Test Fit 2 mm new sketch design from OS 7 1_v1 (Autodesk Fusion 360 design; units mm, degrees)
Autodesk Fusion 360 part; units mm, degrees
(part 1 of 2)
ref_plane "WorkPlane12" through (0, -1, 0) normal (0, 1, 0) x (0, 0, 1)
sketch "MyStock" plane through (0, 0, 0) normal (0, 0, 1) x (1, 0, 0)
  line L0 (-9.525, 182) -> (9.525, 182)
  line L1 (9.525, 182) -> (9.525, 0)
  line L2 (-9.525, 0) -> (-9.525, 182)
  line L3 (-9.525, 0) -> (9.525, 0)
  dimension "d2016" = 9.525
  dimension "d2017" = 9.525
  dimension "d2102" = 182
  constraint horizontal L0
  constraint vertical L1
  constraint vertical L2
  constraint perpendicular L1 L3
  constraint coincident origin L3
  measures "d2016" distance of origin L1
  measures "d2017" distance of origin L2
  measures "d2102" vertical distance of origin L0.end
extrude "Extrude21" add sketch "MyStock" along normal blind 3.175 makes body 1
sketch "Box Big part" plane through (0, 0, 0) normal (0, 0, 1) x (1, 0, 0)
  line L0 (-224.905, 0) -> (-240, 0)
  line L1 (0, 16.095) -> (0, 0)
  line L2 (-240, 0) -> (-224.905, 0)
  line L3 (-224.905, 0) -> (-224.905, 1.5613)
  line L4 (-223.7758, 3.175) -> (-216.2242, 3.175)
  line L5 (-215.095, 1.5613) -> (-215.095, 0)
  line L6 (-240, 16.095) -> (-238.4387, 16.095)
  line L7 (-236.825, 17.2242) -> (-236.825, 24.7758)
  line L8 (-238.4387, 25.905) -> (-240, 25.905)
  line L9 (-215.095, 0) -> (-204.905, 0)
  line L10 (1.75, 0) -> (22.5, 0)
  arc A0 (-215.095, 1.5613) -> (-216.2242, 3.175) centre (-215.5171, 2.4679) ccw
  arc A1 (-223.7758, 3.175) -> (-224.905, 1.5613) centre (-224.4829, 2.4679) ccw
  line L11 (-240, 0) -> (-240, 16.095)
  line L12 (-240, 25.905) -> (-240, 36.095)
  arc A2 (-238.4387, 16.095) -> (-236.825, 17.2242) centre (-237.5321, 16.5171) ccw
  arc A3 (-236.825, 24.7758) -> (-238.4387, 25.905) centre (-237.5321, 25.4829) ccw
  line L13 (-302, 91) -> (0, 91) construction
  line L14 (-120, -20) -> (-120, 200) construction
  arc A4 (-1.5613, 25.905) -> (-3.175, 24.7758) centre (-2.4679, 25.4829) ccw
  arc A5 (-3.175, 17.2242) -> (-1.5613, 16.095) centre (-2.4679, 16.5171) ccw
  line L15 (-3.175, 17.2242) -> (-3.175, 24.7758)
  line L16 (-1.5613, 25.905) -> (0, 25.905)
  line L17 (0, 25.905) -> (0, 36.095)
  line L18 (0, 16.095) -> (-1.5613, 16.095)
  line L19 (0, 16.095) -> (0, 0)
  line L20 (-215.095, 180.4387) -> (-215.095, 182)
  line L21 (-224.905, 182) -> (-224.905, 180.4387)
  line L22 (-215.095, 182) -> (-204.905, 182)
  arc A6 (-216.2242, 178.825) -> (-215.095, 180.4387) centre (-215.5171, 179.5321) ccw
  line L23 (-224.905, 182) -> (-240, 182)
  arc A7 (-224.905, 180.4387) -> (-223.7758, 178.825) centre (-224.4829, 179.5321) ccw
  line L24 (-223.7758, 178.825) -> (-216.2242, 178.825)
  line L25 (-240, 182) -> (-224.905, 182)
  arc A8 (-195.095, 1.5613) -> (-196.2242, 3.175) centre (-195.5171, 2.4679) ccw
  line L26 (-195.095, 1.5613) -> (-195.095, 0)
  arc A9 (-203.7758, 3.175) -> (-204.905, 1.5613) centre (-204.4829, 2.4679) ccw
  line L27 (-195.095, 0) -> (-184.905, 0)
  line L28 (-203.7758, 3.175) -> (-196.2242, 3.175)
  line L29 (-204.905, 0) -> (-204.905, 1.5613)
  arc A10 (-175.095, 1.5613) -> (-176.2242, 3.175) centre (-175.5171, 2.4679) ccw
  line L30 (-175.095, 1.5613) -> (-175.095, 0)
  arc A11 (-183.7758, 3.175) -> (-184.905, 1.5613) centre (-184.4829, 2.4679) ccw
  line L31 (-175.095, 0) -> (-164.905, 0)
  line L32 (-183.7758, 3.175) -> (-176.2242, 3.175)
  line L33 (-184.905, 0) -> (-184.905, 1.5613)
  arc A12 (-155.095, 1.5613) -> (-156.2242, 3.175) centre (-155.5171, 2.4679) ccw
  line L34 (-155.095, 1.5613) -> (-155.095, 0)
  arc A13 (-163.7758, 3.175) -> (-164.905, 1.5613) centre (-164.4829, 2.4679) ccw
  line L35 (-155.095, 0) -> (-144.905, 0)
  line L36 (-163.7758, 3.175) -> (-156.2242, 3.175)
  line L37 (-164.905, 0) -> (-164.905, 1.5613)
  arc A14 (-135.095, 1.5613) -> (-136.2242, 3.175) centre (-135.5171, 2.4679) ccw
  line L38 (-135.095, 1.5613) -> (-135.095, 0)
  arc A15 (-143.7758, 3.175) -> (-144.905, 1.5613) centre (-144.4829, 2.4679) ccw
  line L39 (-135.095, 0) -> (-124.905, 0)
  line L40 (-143.7758, 3.175) -> (-136.2242, 3.175)
  line L41 (-144.905, 0) -> (-144.905, 1.5613)
  arc A16 (-115.095, 1.5613) -> (-116.2242, 3.175) centre (-115.5171, 2.4679) ccw
  line L42 (-115.095, 1.5613) -> (-115.095, 0)
  arc A17 (-123.7758, 3.175) -> (-124.905, 1.5613) centre (-124.4829, 2.4679) ccw
  line L43 (-115.095, 0) -> (-104.905, 0)
  line L44 (-123.7758, 3.175) -> (-116.2242, 3.175)
  line L45 (-124.905, 0) -> (-124.905, 1.5613)
  arc A18 (-95.095, 1.5613) -> (-96.2242, 3.175) centre (-95.5171, 2.4679) ccw
  line L46 (-95.095, 1.5613) -> (-95.095, 0)
  arc A19 (-103.7758, 3.175) -> (-104.905, 1.5613) centre (-104.4829, 2.4679) ccw
  line L47 (-95.095, 0) -> (-84.905, 0)
  line L48 (-103.7758, 3.175) -> (-96.2242, 3.175)
  line L49 (-104.905, 0) -> (-104.905, 1.5613)
  line L50 (0, 0) -> (-4.905, 0)
  line L51 (-238.4387, 45.905) -> (-240, 45.905)
  line L52 (-240, 36.095) -> (-238.4387, 36.095)
  arc A20 (-238.4387, 36.095) -> (-236.825, 37.2242) centre (-237.5321, 36.5171) ccw
  line L53 (-240, 45.905) -> (-240, 56.095)
  arc A21 (-236.825, 44.7758) -> (-238.4387, 45.905) centre (-237.5321, 45.4829) ccw
  line L54 (-236.825, 37.2242) -> (-236.825, 44.7758)
  line L55 (-238.4387, 65.905) -> (-240, 65.905)
  line L56 (-240, 56.095) -> (-238.4387, 56.095)
  arc A22 (-238.4387, 56.095) -> (-236.825, 57.2242) centre (-237.5321, 56.5171) ccw
  line L57 (-240, 65.905) -> (-240, 76.095)
  arc A23 (-236.825, 64.7758) -> (-238.4387, 65.905) centre (-237.5321, 65.4829) ccw
  line L58 (-236.825, 57.2242) -> (-236.825, 64.7758)
  line L59 (-238.4387, 85.905) -> (-240, 85.905)
  line L60 (-240, 76.095) -> (-238.4387, 76.095)
  arc A24 (-238.4387, 76.095) -> (-236.825, 77.2242) centre (-237.5321, 76.5171) ccw
  line L61 (-240, 85.905) -> (-240, 96.095)
  arc A25 (-236.825, 84.7758) -> (-238.4387, 85.905) centre (-237.5321, 85.4829) ccw
  line L62 (-236.825, 77.2242) -> (-236.825, 84.7758)
  line L63 (-238.4387, 105.905) -> (-240, 105.905)
  line L64 (-240, 96.095) -> (-238.4387, 96.095)
  arc A26 (-238.4387, 96.095) -> (-236.825, 97.2242) centre (-237.5321, 96.5171) ccw
  line L65 (-240, 105.905) -> (-240, 116.095)
  arc A27 (-236.825, 104.7758) -> (-238.4387, 105.905) centre (-237.5321, 105.4829) ccw
  line L66 (-236.825, 97.2242) -> (-236.825, 104.7758)
  arc A28 (-196.2242, 178.825) -> (-195.095, 180.4387) centre (-195.5171, 179.5321) ccw
  line L67 (-195.095, 180.4387) -> (-195.095, 182)
  arc A29 (-204.905, 180.4387) -> (-203.7758, 178.825) centre (-204.4829, 179.5321) ccw
  line L68 (-203.7758, 178.825) -> (-196.2242, 178.825)
  line L69 (-204.905, 182) -> (-204.905, 180.4387)
  line L70 (-195.095, 182) -> (-184.905, 182)
  arc A30 (-176.2242, 178.825) -> (-175.095, 180.4387) centre (-175.5171, 179.5321) ccw
  line L71 (-175.095, 180.4387) -> (-175.095, 182)
  arc A31 (-184.905, 180.4387) -> (-183.7758, 178.825) centre (-184.4829, 179.5321) ccw
  line L72 (-183.7758, 178.825) -> (-176.2242, 178.825)
  line L73 (-184.905, 182) -> (-184.905, 180.4387)
  line L74 (-175.095, 182) -> (-164.905, 182)
  arc A32 (-156.2242, 178.825) -> (-155.095, 180.4387) centre (-155.5171, 179.5321) ccw
  line L75 (-155.095, 180.4387) -> (-155.095, 182)
  arc A33 (-164.905, 180.4387) -> (-163.7758, 178.825) centre (-164.4829, 179.5321) ccw
  line L76 (-163.7758, 178.825) -> (-156.2242, 178.825)
  line L77 (-164.905, 182) -> (-164.905, 180.4387)
  line L78 (-155.095, 182) -> (-144.905, 182)
  arc A34 (-136.2242, 178.825) -> (-135.095, 180.4387) centre (-135.5171, 179.5321) ccw
  line L79 (-135.095, 180.4387) -> (-135.095, 182)
  arc A35 (-144.905, 180.4387) -> (-143.7758, 178.825) centre (-144.4829, 179.5321) ccw
  line L80 (-143.7758, 178.825) -> (-136.2242, 178.825)
  line L81 (-144.905, 182) -> (-144.905, 180.4387)
  line L82 (-135.095, 182) -> (-124.905, 182)
  arc A36 (-116.2242, 178.825) -> (-115.095, 180.4387) centre (-115.5171, 179.5321) ccw
  line L83 (-115.095, 180.4387) -> (-115.095, 182)
  arc A37 (-124.905, 180.4387) -> (-123.7758, 178.825) centre (-124.4829, 179.5321) ccw
  line L84 (-123.7758, 178.825) -> (-116.2242, 178.825)
  line L85 (-124.905, 182) -> (-124.905, 180.4387)
  line L86 (-115.095, 182) -> (-104.905, 182)
  arc A38 (-96.2242, 178.825) -> (-95.095, 180.4387) centre (-95.5171, 179.5321) ccw
  line L87 (-95.095, 180.4387) -> (-95.095, 182)
  arc A39 (-104.905, 180.4387) -> (-103.7758, 178.825) centre (-104.4829, 179.5321) ccw
  line L88 (-103.7758, 178.825) -> (-96.2242, 178.825)
  line L89 (-104.905, 182) -> (-104.905, 180.4387)
  line L90 (-95.095, 182) -> (-84.905, 182)
  line L91 (0, 182) -> (-4.905, 182)
  line L92 (-3.175, 37.2242) -> (-3.175, 44.7758)
  line L93 (-1.5613, 45.905) -> (0, 45.905)
  line L94 (0, 45.905) -> (0, 56.095)
  arc A40 (-1.5613, 45.905) -> (-3.175, 44.7758) centre (-2.4679, 45.4829) ccw
  line L95 (0, 36.095) -> (-1.5613, 36.095)
  line L96 (-3.175, 57.2242) -> (-3.175, 64.7758)
  line L97 (-1.5613, 65.905) -> (0, 65.905)
  line L98 (0, 65.905) -> (0, 76.095)
  arc A41 (-1.5613, 65.905) -> (-3.175, 64.7758) centre (-2.4679, 65.4829) ccw
  line L99 (0, 56.095) -> (-1.5613, 56.095)
  line L100 (-3.175, 77.2242) -> (-3.175, 84.7758)
  line L101 (-1.5613, 85.905) -> (0, 85.905)
  line L102 (0, 85.905) -> (0, 96.095)
  arc A42 (-1.5613, 85.905) -> (-3.175, 84.7758) centre (-2.4679, 85.4829) ccw
  line L103 (0, 76.095) -> (-1.5613, 76.095)
  line L104 (-3.175, 97.2242) -> (-3.175, 104.7758)
  line L105 (-1.5613, 105.905) -> (0, 105.905)
  line L106 (0, 105.905) -> (0, 116.095)
  arc A43 (-1.5613, 105.905) -> (-3.175, 104.7758) centre (-2.4679, 105.4829) ccw
  line L107 (0, 96.095) -> (-1.5613, 96.095)
  arc A44 (-3.175, 37.2242) -> (-1.5613, 36.095) centre (-2.4679, 36.5171) ccw
  arc A45 (-3.175, 57.2242) -> (-1.5613, 56.095) centre (-2.4679, 56.5171) ccw
  arc A46 (-3.175, 77.2242) -> (-1.5613, 76.095) centre (-2.4679, 76.5171) ccw
  arc A47 (-3.175, 97.2242) -> (-1.5613, 96.095) centre (-2.4679, 96.5171) ccw
  line L108 (0, 182) -> (0, 176.095)
  line L109 (-240, 182) -> (-240, 176.095)
  arc A48 (-75.095, 1.5613) -> (-76.2242, 3.175) centre (-75.5171, 2.4679) ccw
  line L110 (-75.095, 1.5613) -> (-75.095, 0)
  arc A49 (-83.7758, 3.175) -> (-84.905, 1.5613) centre (-84.4829, 2.4679) ccw
  line L111 (-75.095, 0) -> (-64.905, 0)
  line L112 (-83.7758, 3.175) -> (-76.2242, 3.175)
  line L113 (-84.905, 0) -> (-84.905, 1.5613)
  arc A50 (-55.095, 1.5613) -> (-56.2242, 3.175) centre (-55.5171, 2.4679) ccw
  line L114 (-55.095, 1.5613) -> (-55.095, 0)
  arc A51 (-63.7758, 3.175) -> (-64.905, 1.5613) centre (-64.4829, 2.4679) ccw
  line L115 (-55.095, 0) -> (-44.905, 0)
  line L116 (-63.7758, 3.175) -> (-56.2242, 3.175)
  line L117 (-64.905, 0) -> (-64.905, 1.5613)
  arc A52 (-35.095, 1.5613) -> (-36.2242, 3.175) centre (-35.5171, 2.4679) ccw
  line L118 (-35.095, 1.5613) -> (-35.095, 0)
  arc A53 (-43.7758, 3.175) -> (-44.905, 1.5613) centre (-44.4829, 2.4679) ccw
  line L119 (-35.095, 0) -> (-24.905, 0)
  line L120 (-43.7758, 3.175) -> (-36.2242, 3.175)
  line L121 (-44.905, 0) -> (-44.905, 1.5613)
  arc A54 (-15.095, 1.5613) -> (-16.2242, 3.175) centre (-15.5171, 2.4679) ccw
  line L122 (-15.095, 1.5613) -> (-15.095, 0)
  arc A55 (-23.7758, 3.175) -> (-24.905, 1.5613) centre (-24.4829, 2.4679) ccw
  line L123 (-15.095, 0) -> (-4.905, 0)
  line L124 (-23.7758, 3.175) -> (-16.2242, 3.175)
  line L125 (-24.905, 0) -> (-24.905, 1.5613)
  line L126 (-238.4387, 125.905) -> (-240, 125.905)
  line L127 (-240, 116.095) -> (-238.4387, 116.095)
  arc A56 (-238.4387, 116.095) -> (-236.825, 117.2242) centre (-237.5321, 116.5171) ccw
  line L128 (-240, 125.905) -> (-240, 136.095)
  arc A57 (-236.825, 124.7758) -> (-238.4387, 125.905) centre (-237.5321, 125.4829) ccw
  line L129 (-236.825, 117.2242) -> (-236.825, 124.7758)
  line L130 (-238.4387, 145.905) -> (-240, 145.905)
  line L131 (-240, 136.095) -> (-238.4387, 136.095)
  arc A58 (-238.4387, 136.095) -> (-236.825, 137.2242) centre (-237.5321, 136.5171) ccw
  line L132 (-240, 145.905) -> (-240, 156.095)
  arc A59 (-236.825, 144.7758) -> (-238.4387, 145.905) centre (-237.5321, 145.4829) ccw
  line L133 (-236.825, 137.2242) -> (-236.825, 144.7758)
  line L134 (-238.4387, 165.905) -> (-240, 165.905)
  line L135 (-240, 156.095) -> (-238.4387, 156.095)
  arc A60 (-238.4387, 156.095) -> (-236.825, 157.2242) centre (-237.5321, 156.5171) ccw
  line L136 (-240, 165.905) -> (-240, 176.095)
  arc A61 (-236.825, 164.7758) -> (-238.4387, 165.905) centre (-237.5321, 165.4829) ccw
  line L137 (-236.825, 157.2242) -> (-236.825, 164.7758)
  arc A62 (-76.2242, 178.825) -> (-75.095, 180.4387) centre (-75.5171, 179.5321) ccw
  line L138 (-75.095, 180.4387) -> (-75.095, 182)
  arc A63 (-84.905, 180.4387) -> (-83.7758, 178.825) centre (-84.4829, 179.5321) ccw
  line L139 (-83.7758, 178.825) -> (-76.2242, 178.825)
  line L140 (-84.905, 182) -> (-84.905, 180.4387)
  line L141 (-75.095, 182) -> (-64.905, 182)
  arc A64 (-56.2242, 178.825) -> (-55.095, 180.4387) centre (-55.5171, 179.5321) ccw
  line L142 (-55.095, 180.4387) -> (-55.095, 182)
  arc A65 (-64.905, 180.4387) -> (-63.7758, 178.825) centre (-64.4829, 179.5321) ccw
  line L143 (-63.7758, 178.825) -> (-56.2242, 178.825)
  line L144 (-64.905, 182) -> (-64.905, 180.4387)
  line L145 (-55.095, 182) -> (-44.905, 182)
  arc A66 (-36.2242, 178.825) -> (-35.095, 180.4387) centre (-35.5171, 179.5321) ccw
  line L146 (-35.095, 180.4387) -> (-35.095, 182)
  arc A67 (-44.905, 180.4387) -> (-43.7758, 178.825) centre (-44.4829, 179.5321) ccw
  line L147 (-43.7758, 178.825) -> (-36.2242, 178.825)
  line L148 (-44.905, 182) -> (-44.905, 180.4387)
  line L149 (-35.095, 182) -> (-24.905, 182)
  arc A68 (-16.2242, 178.825) -> (-15.095, 180.4387) centre (-15.5171, 179.5321) ccw
  line L150 (-15.095, 180.4387) -> (-15.095, 182)
  arc A69 (-24.905, 180.4387) -> (-23.7758, 178.825) centre (-24.4829, 179.5321) ccw
  line L151 (-23.7758, 178.825) -> (-16.2242, 178.825)
  line L152 (-24.905, 182) -> (-24.905, 180.4387)
  line L153 (-15.095, 182) -> (-4.905, 182)
  line L154 (-3.175, 117.2242) -> (-3.175, 124.7758)
  line L155 (-1.5613, 125.905) -> (0, 125.905)
  line L156 (0, 125.905) -> (0, 136.095)
  arc A70 (-1.5613, 125.905) -> (-3.175, 124.7758) centre (-2.4679, 125.4829) ccw
  line L157 (0, 116.095) -> (-1.5613, 116.095)
  arc A71 (-3.175, 117.2242) -> (-1.5613, 116.095) centre (-2.4679, 116.5171) ccw
  line L158 (-3.175, 137.2242) -> (-3.175, 144.7758)
  line L159 (-1.5613, 145.905) -> (0, 145.905)
  line L160 (0, 145.905) -> (0, 156.095)
  arc A72 (-1.5613, 145.905) -> (-3.175, 144.7758) centre (-2.4679, 145.4829) ccw
  line L161 (0, 136.095) -> (-1.5613, 136.095)
  arc A73 (-3.175, 137.2242) -> (-1.5613, 136.095) centre (-2.4679, 136.5171) ccw
  line L162 (-3.175, 157.2242) -> (-3.175, 164.7758)
  line L163 (-1.5613, 165.905) -> (0, 165.905)
  line L164 (0, 165.905) -> (0, 176.095)
  arc A74 (-1.5613, 165.905) -> (-3.175, 164.7758) centre (-2.4679, 165.4829) ccw
  line L165 (0, 156.095) -> (-1.5613, 156.095)
  arc A75 (-3.175, 157.2242) -> (-1.5613, 156.095) centre (-2.4679, 156.5171) ccw
  dimension "d34" = 2
  dimension "d36" = 0.4221
  dimension "d37" = 0.7071
  dimension "d38" = 0.4221
  dimension "d48" = 2
  dimension "d49" = 0.4221
  dimension "d50" = 16.095
  dimension "d52" = 0.4221
  dimension "d54" = 0.7071
  dimension "d55" = 9.81
  dimension "d189" = 15.095
  dimension "d473" = 240
  dimension "d2062" = 10.19
  dimension "d2063" = 9.81
  dimension "d2064" = 3.175
  dimension "d2068" = 3.175
  dimension "d2069" = 10.19
  dimension "d2071" = 120
  dimension "d2074" = 20
  dimension "d2075" = 0
  dimension "d2076" = 4.905
  dimension "d2080" = 0
  dimension "d2081" = 20
  dimension "d2084" = 20
  dimension "d2085" = 0
  dimension "d2087" = 4.905
  dimension "d2088" = 182
  dimension "d2091" = 0
  dimension "d2092" = 20
  dimension "d2095" = 5.905
  dimension "d2097" = 5.905
  dimension "d2098" = 182
  dimension "d2103" = 91
  constraint horizontal L0
  constraint vertical L11
  constraint vertical L1
  constraint coincident L1.end L19.end
  constraint horizontal L2
  constraint perpendicular L2 L3
  constraint perpendicular L3 L4
  constraint perpendicular L4 L5
  constraint equal A0 A1
  constraint horizontal A1.centre A0.centre
  constraint perpendicular L6 L11
  constraint perpendicular L6 L7
  constraint perpendicular L8 L11
  constraint equal A2 A3
  constraint vertical A3.centre A2.centre
  constraint perpendicular L5 L9
  constraint collinear L0 L10
  constraint collinear L9 L10
  constraint perpendicular L8 L12
  constraint collinear L11 L12
  constraint perpendicular L1 L13
  constraint symmetric L6.start L14 L1.start
  constraint symmetric L8.end L14 L16.end
  constraint symmetric L12.end L14 L17.end
  constraint symmetric L7.start L14 A5.start
  constraint symmetric L6.end L14 A5.end
  constraint symmetric A2 L14 A5
  constraint symmetric L8.start L14 A4.start
  constraint symmetric L7.end L14 A4.end
  constraint symmetric A3 L14 A4
  constraint symmetric L0.end L13 L23.end
  constraint symmetric L0.start L13 L21.start
  constraint symmetric L5.end L13 L20.end
  constraint symmetric L9.end L13 L22.end
  constraint symmetric L5.start L13 L20.start
  constraint symmetric L3.end L13 L21.end
  constraint symmetric L4.end L13 A6.start
  constraint symmetric A0 L13 A6
  constraint symmetric L4.start L13 A7.end
  constraint symmetric A1 L13 A7
  constraint perpendicular L19 L50
  constraint horizontal L91
  constraint perpendicular L91 L108
  constraint vertical L109
  constraint collinear L11 L109
  constraint collinear L19 L108
  measures "d34" diameter of A1
  measures "d36" distance of L3 A1.centre
  measures "d37" distance of L4 A1.centre
  measures "d38" horizontal distance of L5.end A0.centre
  measures "d48" diameter of A3
  measures "d49" distance of L6 A2.centre
  measures "d50" distance of L2 L6
  measures "d52" distance of L8 A3.centre
  measures "d54" distance of L7 A2.centre
  measures "d55" distance of L6 L8
  measures "d189" distance of L3 L11
  measures "d473" distance of L1 L11
  measures "d2062" distance of L5.end L9.end
  measures "d2063" distance of L5 L3.end
  measures "d2064" distance of L0 L4
  measures "d2068" distance of L7 L11
  measures "d2069" distance of L8.end L12.end
  measures "d2071" distance of L1.end L14
  measures "d2076" distance of L1.end L50.end
  measures "d2087" distance of L91.start L91.end
  measures "d2088" distance of L1.end L91.start
  measures "d2095" distance of L91.start L108.end
  measures "d2097" distance of L23.end L109.end
  measures "d2098" distance of L10 L23.end
  measures "d2103" distance of L1.end L13
sketch "Box Medium part" plane through (0, 0, 0) normal (0, 0, 1) x (1, 0, 0)
  line L0 (28.2242, 3.175) -> (35.7758, 3.175)
  line L1 (240.4387, 14.905) -> (242, 14.905)
  line L2 (238.825, 3.175) -> (238.825, 13.7758)
  line L3 (242, 25.095) -> (240.4387, 25.095)
  line L4 (2, 60) -> (242, 60) construction
  line L5 (27.095, 0) -> (27.095, 1.5613)
  line L6 (240.4387, 34.905) -> (242, 34.905)
  line L7 (5.175, 3.175) -> (15.7758, 3.175)
  line L8 (36.905, 1.5613) -> (36.905, 0)
  line L9 (242, 60) -> (242, 0) construction
  line L10 (238.825, 26.2242) -> (238.825, 33.7758)
  line L11 (16.905, 1.5613) -> (16.905, 0)
  line L12 (2, -28) -> (2, 0) construction
  arc A0 (16.905, 1.5613) -> (15.7758, 3.175) centre (16.4829, 2.4679) ccw
  arc A1 (28.2242, 3.175) -> (27.095, 1.5613) centre (27.5171, 2.4679) ccw
  arc A2 (36.905, 1.5613) -> (35.7758, 3.175) centre (36.4829, 2.4679) ccw
  arc A3 (240.4387, 14.905) -> (238.825, 13.7758) centre (239.5321, 14.4829) ccw
  line L13 (16.905, 0) -> (27.095, 0)
  line L14 (-22, 30) -> (297, 30) construction
  line L15 (122, -24.8824) -> (122, 81) construction
  arc A4 (238.825, 26.2242) -> (240.4387, 25.095) centre (239.5321, 25.5171) ccw
  arc A5 (240.4387, 34.905) -> (238.825, 33.7758) centre (239.5321, 34.4829) ccw
  line L16 (36.905, 0) -> (47.095, 0)
  line L17 (242, 34.905) -> (242, 45.095)
  line L18 (2, -28) -> (2, 30) construction
  line L19 (2, 60) -> (2, 30) construction
  line L20 (0, 0) -> (47.095, 0) construction
  line L21 (122, 0) -> (242, 0) construction
  line L22 (36.905, 58.4387) -> (36.905, 60)
  arc A6 (35.7758, 56.825) -> (36.905, 58.4387) centre (36.4829, 57.5321) ccw
  line L23 (36.905, 60) -> (47.095, 60)
  arc A7 (15.7758, 56.825) -> (16.905, 58.4387) centre (16.4829, 57.5321) ccw
  line L24 (27.095, 60) -> (27.095, 58.4387)
  line L25 (16.905, 58.4387) -> (16.905, 60)
  arc A8 (27.095, 58.4387) -> (28.2242, 56.825) centre (27.5171, 57.5321) ccw
  line L26 (16.905, 60) -> (27.095, 60)
  line L27 (28.2242, 56.825) -> (35.7758, 56.825)
  line L28 (0, 60) -> (47.095, 60) construction
  line L29 (5.175, 56.825) -> (15.7758, 56.825)
  line L30 (3.5613, 14.905) -> (2, 14.905)
  arc A9 (5.175, 33.7758) -> (3.5613, 34.905) centre (4.4679, 34.4829) ccw
  line L31 (5.175, 3.175) -> (5.175, 13.7758)
  line L32 (3.5613, 34.905) -> (2, 34.905)
  line L33 (5.175, 26.2242) -> (5.175, 33.7758)
  line L34 (2, 25.095) -> (3.5613, 25.095)
  arc A10 (5.175, 13.7758) -> (3.5613, 14.905) centre (4.4679, 14.4829) ccw
  arc A11 (3.5613, 25.095) -> (5.175, 26.2242) centre (4.4679, 25.5171) ccw
  line L35 (2, 34.905) -> (2, 45.095)
  arc A12 (56.905, 1.5613) -> (55.7758, 3.175) centre (56.4829, 2.4679) ccw
  line L36 (48.2242, 3.175) -> (55.7758, 3.175)
  arc A13 (48.2242, 3.175) -> (47.095, 1.5613) centre (47.5171, 2.4679) ccw
  line L37 (56.905, 0) -> (67.095, 0)
  line L38 (56.905, 1.5613) -> (56.905, 0)
  line L39 (47.095, 0) -> (47.095, 1.5613)
  arc A14 (76.905, 1.5613) -> (75.7758, 3.175) centre (76.4829, 2.4679) ccw
  line L40 (68.2242, 3.175) -> (75.7758, 3.175)
  arc A15 (68.2242, 3.175) -> (67.095, 1.5613) centre (67.5171, 2.4679) ccw
  line L41 (76.905, 0) -> (87.095, 0)
  line L42 (76.905, 1.5613) -> (76.905, 0)
  line L43 (67.095, 0) -> (67.095, 1.5613)
  arc A16 (96.905, 1.5613) -> (95.7758, 3.175) centre (96.4829, 2.4679) ccw
  line L44 (88.2242, 3.175) -> (95.7758, 3.175)
  arc A17 (88.2242, 3.175) -> (87.095, 1.5613) centre (87.5171, 2.4679) ccw
  line L45 (96.905, 0) -> (107.095, 0)
  line L46 (96.905, 1.5613) -> (96.905, 0)
  line L47 (87.095, 0) -> (87.095, 1.5613)
  arc A18 (116.905, 1.5613) -> (115.7758, 3.175) centre (116.4829, 2.4679) ccw
  line L48 (108.2242, 3.175) -> (115.7758, 3.175)
  arc A19 (108.2242, 3.175) -> (107.095, 1.5613) centre (107.5171, 2.4679) ccw
  line L49 (116.905, 0) -> (127.095, 0)
  line L50 (116.905, 1.5613) -> (116.905, 0)
  line L51 (107.095, 0) -> (107.095, 1.5613)
  arc A20 (136.905, 1.5613) -> (135.7758, 3.175) centre (136.4829, 2.4679) ccw
  line L52 (128.2242, 3.175) -> (135.7758, 3.175)
  arc A21 (128.2242, 3.175) -> (127.095, 1.5613) centre (127.5171, 2.4679) ccw
  line L53 (136.905, 0) -> (147.095, 0)
  line L54 (136.905, 1.5613) -> (136.905, 0)
  line L55 (127.095, 0) -> (127.095, 1.5613)
  line L56 (47.095, 60) -> (47.095, 58.4387)
  line L57 (48.2242, 56.825) -> (55.7758, 56.825)
  arc A22 (55.7758, 56.825) -> (56.905, 58.4387) centre (56.4829, 57.5321) ccw
  arc A23 (47.095, 58.4387) -> (48.2242, 56.825) centre (47.5171, 57.5321) ccw
  line L58 (56.905, 60) -> (67.095, 60)
  line L59 (56.905, 58.4387) -> (56.905, 60)
  line L60 (67.095, 60) -> (67.095, 58.4387)
  line L61 (68.2242, 56.825) -> (75.7758, 56.825)
  arc A24 (75.7758, 56.825) -> (76.905, 58.4387) centre (76.4829, 57.5321) ccw
  arc A25 (67.095, 58.4387) -> (68.2242, 56.825) centre (67.5171, 57.5321) ccw
  line L62 (76.905, 60) -> (87.095, 60)
  line L63 (76.905, 58.4387) -> (76.905, 60)
  line L64 (87.095, 60) -> (87.095, 58.4387)
  line L65 (88.2242, 56.825) -> (95.7758, 56.825)
  arc A26 (95.7758, 56.825) -> (96.905, 58.4387) centre (96.4829, 57.5321) ccw
  arc A27 (87.095, 58.4387) -> (88.2242, 56.825) centre (87.5171, 57.5321) ccw
  line L66 (96.905, 60) -> (107.095, 60)
  line L67 (96.905, 58.4387) -> (96.905, 60)
  line L68 (107.095, 60) -> (107.095, 58.4387)
  line L69 (108.2242, 56.825) -> (115.7758, 56.825)
  arc A28 (115.7758, 56.825) -> (116.905, 58.4387) centre (116.4829, 57.5321) ccw
  arc A29 (107.095, 58.4387) -> (108.2242, 56.825) centre (107.5171, 57.5321) ccw
  line L70 (116.905, 60) -> (127.095, 60)
  line L71 (116.905, 58.4387) -> (116.905, 60)
  line L72 (127.095, 60) -> (127.095, 58.4387)
  line L73 (128.2242, 56.825) -> (135.7758, 56.825)
  arc A30 (135.7758, 56.825) -> (136.905, 58.4387) centre (136.4829, 57.5321) ccw
  arc A31 (127.095, 58.4387) -> (128.2242, 56.825) centre (127.5171, 57.5321) ccw
  line L74 (136.905, 60) -> (147.095, 60)
  line L75 (136.905, 58.4387) -> (136.905, 60)
  line L76 (227.095, 1.5613) -> (227.095, 0)
  arc A32 (228.2242, 3.175) -> (227.095, 1.5613) centre (227.5171, 2.4679) ccw
  line L77 (238.825, 3.175) -> (228.2242, 3.175)
  line L78 (242, 88) -> (242, 60) construction
  line L79 (227.095, 58.4387) -> (227.095, 60)
  line L80 (242, 60) -> (242, 30) construction
  arc A33 (227.095, 58.4387) -> (228.2242, 56.825) centre (227.5171, 57.5321) ccw
  line L81 (238.825, 56.825) -> (228.2242, 56.825)
  line L82 (2, 14.905) -> (2, 25.095)
  arc A34 (3.5613, 45.095) -> (5.175, 46.2242) centre (4.4679, 45.5171) ccw
  line L83 (3.5613, 45.095) -> (2, 45.095)
  line L84 (5.175, 56.825) -> (5.175, 46.2242)
  arc A35 (238.825, 46.2242) -> (240.4387, 45.095) centre (239.5321, 45.5171) ccw
  line L85 (240.4387, 45.095) -> (242, 45.095)
  line L86 (238.825, 56.825) -> (238.825, 46.2242)
  line L87 (242, 25.095) -> (242, 14.905)
  arc A36 (156.905, 1.5613) -> (155.7758, 3.175) centre (156.4829, 2.4679) ccw
  line L88 (148.2242, 3.175) -> (155.7758, 3.175)
  arc A37 (148.2242, 3.175) -> (147.095, 1.5613) centre (147.5171, 2.4679) ccw
  line L89 (156.905, 0) -> (167.095, 0)
  line L90 (156.905, 1.5613) -> (156.905, 0)
  line L91 (147.095, 0) -> (147.095, 1.5613)
  arc A38 (176.905, 1.5613) -> (175.7758, 3.175) centre (176.4829, 2.4679) ccw
  line L92 (168.2242, 3.175) -> (175.7758, 3.175)
  arc A39 (168.2242, 3.175) -> (167.095, 1.5613) centre (167.5171, 2.4679) ccw
  line L93 (176.905, 0) -> (187.095, 0)
  line L94 (176.905, 1.5613) -> (176.905, 0)
  line L95 (167.095, 0) -> (167.095, 1.5613)
  arc A40 (196.905, 1.5613) -> (195.7758, 3.175) centre (196.4829, 2.4679) ccw
  line L96 (188.2242, 3.175) -> (195.7758, 3.175)
  arc A41 (188.2242, 3.175) -> (187.095, 1.5613) centre (187.5171, 2.4679) ccw
  line L97 (196.905, 0) -> (207.095, 0)
  line L98 (196.905, 1.5613) -> (196.905, 0)
  line L99 (187.095, 0) -> (187.095, 1.5613)
  arc A42 (216.905, 1.5613) -> (215.7758, 3.175) centre (216.4829, 2.4679) ccw
  line L100 (208.2242, 3.175) -> (215.7758, 3.175)
  arc A43 (208.2242, 3.175) -> (207.095, 1.5613) centre (207.5171, 2.4679) ccw
  line L101 (216.905, 0) -> (227.095, 0)
  line L102 (216.905, 1.5613) -> (216.905, 0)
  line L103 (207.095, 0) -> (207.095, 1.5613)
  line L104 (147.095, 60) -> (147.095, 58.4387)
  line L105 (148.2242, 56.825) -> (155.7758, 56.825)
  arc A44 (155.7758, 56.825) -> (156.905, 58.4387) centre (156.4829, 57.5321) ccw
  arc A45 (147.095, 58.4387) -> (148.2242, 56.825) centre (147.5171, 57.5321) ccw
  line L106 (156.905, 60) -> (167.095, 60)
  line L107 (156.905, 58.4387) -> (156.905, 60)
  line L108 (167.095, 60) -> (167.095, 58.4387)
  line L109 (168.2242, 56.825) -> (175.7758, 56.825)
  arc A46 (175.7758, 56.825) -> (176.905, 58.4387) centre (176.4829, 57.5321) ccw
  arc A47 (167.095, 58.4387) -> (168.2242, 56.825) centre (167.5171, 57.5321) ccw
  line L110 (176.905, 60) -> (187.095, 60)
  line L111 (176.905, 58.4387) -> (176.905, 60)
  line L112 (187.095, 60) -> (187.095, 58.4387)
  line L113 (188.2242, 56.825) -> (195.7758, 56.825)
  arc A48 (195.7758, 56.825) -> (196.905, 58.4387) centre (196.4829, 57.5321) ccw
  arc A49 (187.095, 58.4387) -> (188.2242, 56.825) centre (187.5171, 57.5321) ccw
  line L114 (196.905, 60) -> (207.095, 60)
  line L115 (196.905, 58.4387) -> (196.905, 60)
  line L116 (207.095, 60) -> (207.095, 58.4387)
  line L117 (208.2242, 56.825) -> (215.7758, 56.825)
  arc A50 (215.7758, 56.825) -> (216.905, 58.4387) centre (216.4829, 57.5321) ccw
  arc A51 (207.095, 58.4387) -> (208.2242, 56.825) centre (207.5171, 57.5321) ccw
  line L118 (216.905, 60) -> (227.095, 60)
  line L119 (216.905, 58.4387) -> (216.905, 60)
  point P0 (0, 60)
  point P1 (0, 60)
  point P2 (0, 60)
  point P3 (0, 60)
  point P4 (0, 60)
  point P5 (244, 60)
  point P6 (244, 60)
  point P7 (244, 60)
  point P8 (244, 60)
  point P9 (244, 60)
  point P10 (244, 60)
  dimension "d1829" = 60
  dimension "d1833" = 240
  dimension "d1834" = 2
  dimension "d1835" = 0.4221
  dimension "d1836" = 0.7071
  dimension "d1837" = 0.4221
  dimension "d1842" = 2
  dimension "d1843" = 0.7071
  dimension "d1844" = 0.4221
  dimension "d1845" = 2
  dimension "d1846" = 0.4221
  dimension "d1848" = 2
  dimension "d1849" = 0.4221
  dimension "d1850" = 10.19
  dimension "d1862" = 0.4221
  dimension "d2106" = 14.905
  dimension "d2107" = 2
  dimension "d2109" = 9.81
  dimension "d2110" = 10.19
  dimension "d2111" = 30
  dimension "d2112" = 122
  dimension "d2113" = 58
  dimension "d2114" = 242
  dimension "d2115" = 3.175
  dimension "d2116" = 3.175
  dimension "d2117" = 9.81
  dimension "d2118" = 10.19
  dimension "d2119" = 10.19
  dimension "d2122" = 11.73
  dimension "d2123" = 3.175
  dimension "d2126" = 20
  dimension "d2127" = 0
  dimension "d2130" = 20
  dimension "d2131" = 0
  dimension "d2134" = 0
  dimension "d2135" = 20
  dimension "d2138" = 0
  dimension "d2139" = 20
  constraint horizontal L4
  constraint vertical L9
  constraint perpendicular L0 L5
  constraint perpendicular L0 L8
  constraint equal A1 A2
  constraint horizontal A2.centre A1.centre
  constraint coincident L1.end L9
  constraint perpendicular L1 L9
  constraint horizontal L3
  constraint vertical L10
  constraint horizontal L6
  constraint coincident L3.start L9
  constraint equal A4 A5
  constraint vertical A5.centre A4.centre
  constraint vertical A5.centre A3.centre
  constraint horizontal A0.centre A1.centre
  constraint collinear L0 L7
  constraint collinear L5.start L11.end L20.start
  constraint perpendicular L5 L13
  constraint horizontal L13
  constraint parallel L4 L14
  constraint vertical L15
  constraint perpendicular L14 L18
  constraint horizontal L20
  constraint coincident L20.start origin
  constraint collinear L13 L20
  constraint coincident L9.end L21.end
  constraint collinear L2 L10
  constraint perpendicular L8 L16
  constraint coincident L9 L17.end
  constraint perpendicular L6 L17
  constraint coincident L14 L18.end
  constraint collinear L18 L19
  constraint coincident L15 L21.start
  constraint collinear L20 L21
  constraint symmetric L20.start L14 P4
  constraint symmetric L8.end L14 L22.end
  constraint symmetric L5.start L14 L24.start
  constraint symmetric L11.end L14 L25.end
  constraint symmetric L7.end L14 A7.start
  constraint symmetric L11.start L14 A7.end
  constraint symmetric A0 L14 A7
  constraint symmetric L5.end L14 L24.end
  constraint symmetric L0.start L14 A8.end
  constraint symmetric A1 L14 A8
  constraint symmetric L0.end L14 A6.start
  constraint symmetric L8.start L14 L22.start
  constraint symmetric A2 L14 A6
  constraint symmetric L14 L20.start P4
  constraint symmetric L14 L16.end L23.end
  constraint symmetric L14 L7.start L29.start
  constraint symmetric L1.end L15 L30.end
  constraint symmetric L6.end L15 L32.end
  constraint symmetric L3.start L15 L34.start
  constraint symmetric L2.end L15 L31.end
  constraint symmetric L1.start L15 L30.start
  constraint symmetric A3 L15 A10
  constraint symmetric L15 L3.end L34.end
  constraint symmetric L15 L10.start L33.start
  constraint symmetric L15 A4 A11
  constraint symmetric L15 L10.end A9.start
  constraint symmetric L15 L6.start A9.end
  constraint symmetric L15 A5 A9
  constraint symmetric L15 L17.end L35.end
  constraint symmetric L15 L2.start L7.start
  constraint symmetric L11.end L15 L76.end
  constraint symmetric L7.end L15 A32.start
  constraint symmetric L11.start L15 L76.start
  constraint symmetric A0 L15 A32
  constraint symmetric L15 L7.start L2.start
  constraint symmetric L4.start L15 L4.end
  constraint symmetric L15 L18.end L80.end
  constraint symmetric L15 A7.end L79.start
  constraint symmetric L15 P4 P10
  constraint symmetric L15 L25.end L79.end
  constraint symmetric L15 A7.start A33.end
  constraint symmetric L15 L29.start L81.start
  constraint symmetric L15 A7 A33
  constraint perpendicular L34 L82
  constraint symmetric L14 L30.end L35.end
  constraint symmetric L14 L31.end A34.end
  constraint symmetric L14 L30.start A34.start
  constraint symmetric L14 A10 A34
  constraint symmetric L1.end L14 L17.end
  constraint symmetric L2.end L14 A35.start
  constraint symmetric L1.start L14 A35.end
  constraint symmetric A3 L14 A35
  constraint symmetric L14 L2.start L81.start
  constraint coincident L18.end L19.end
  measures "d1829" distance of L4.end L9.end
  measures "d1833" distance of L4.start L4.end
  measures "d1834" diameter of A1
  measures "d1835" distance of A1.centre L5
  measures "d1836" distance of A1.centre L0
  measures "d1837" horizontal distance of L8.end A2.centre
  measures "d1842" diameter of A4
  measures "d1843" distance of A4.centre L10
  measures "d1844" distance of A4.centre L3
  measures "d1845" diameter of A3
  measures "d1846" distance of A3.centre L1
  measures "d1848" diameter of A0
  measures "d1849" distance of A0.centre L11
  measures "d1850" distance of L1 L3
  measures "d1862" distance of A5.centre L6
  measures "d2106" distance of L11 L12
  measures "d2107" horizontal distance of L20.start L12.end
  measures "d2109" distance of L5 L8
  measures "d2110" distance of L5 L11
  measures "d2111" distance of L14 L20.start
  measures "d2112" distance of L20.start L15
  measures "d2113" distance of L12.start L18.end
  measures "d2114" distance of L20.start L9.end
  measures "d2115" distance of L7 L20
  measures "d2116" distance of L2 L9
  measures "d2117" distance of L3 L6.start
  measures "d2118" distance of L8.end L16.end
  measures "d2119" distance of L6.end L17.end
  measures "d2122" vertical distance of L1.start L2.start
  measures "d2123" distance of L2.start L20
sketch "Box Small Part" plane through (0, 0, 0) normal (0, 0, 1) x (1, 0, 0)
  line L0 (-286.905, 0) -> (-286.905, 1.5613)
  line L1 (-245.175, 0) -> (-245.175, 14.7758)
  line L2 (-243.5613, 35.905) -> (-242, 35.905)
  line L3 (-285.7758, 3.175) -> (-278.2242, 3.175)
  line L4 (-277.095, 1.5613) -> (-277.095, 0)
  line L5 (-243.5613, 15.905) -> (-242, 15.905)
  line L6 (-242, 26.095) -> (-242, 15.905)
  arc A0 (-243.5613, 15.905) -> (-245.175, 14.7758) centre (-244.4679, 15.4829) ccw
  arc A1 (-245.175, 27.2242) -> (-243.5613, 26.095) centre (-244.4679, 26.5171) ccw
  line L7 (-242, 26.095) -> (-243.5613, 26.095)
  line L8 (-245.175, 27.2242) -> (-245.175, 34.7758)
  arc A2 (-243.5613, 35.905) -> (-245.175, 34.7758) centre (-244.4679, 35.4829) ccw
  line L9 (-266.905, 0) -> (-277.095, 0)
  arc A3 (-285.7758, 3.175) -> (-286.905, 1.5613) centre (-286.4829, 2.4679) ccw
  arc A4 (-277.095, 1.5613) -> (-278.2242, 3.175) centre (-277.5171, 2.4679) ccw
  line L10 (-242, 46.095) -> (-242, 35.905)
  line L11 (-242, 66.095) -> (-242, 55.905)
  line L12 (-245.175, 47.2242) -> (-245.175, 54.7758)
  line L13 (-242, 46.095) -> (-243.5613, 46.095)
  line L14 (-243.5613, 55.905) -> (-242, 55.905)
  arc A5 (-245.175, 47.2242) -> (-243.5613, 46.095) centre (-244.4679, 46.5171) ccw
  arc A6 (-243.5613, 55.905) -> (-245.175, 54.7758) centre (-244.4679, 55.4829) ccw
  line L15 (-242, 86.095) -> (-242, 75.905)
  line L16 (-245.175, 67.2242) -> (-245.175, 74.7758)
  line L17 (-242, 66.095) -> (-243.5613, 66.095)
  line L18 (-243.5613, 75.905) -> (-242, 75.905)
  arc A7 (-245.175, 67.2242) -> (-243.5613, 66.095) centre (-244.4679, 66.5171) ccw
  arc A8 (-243.5613, 75.905) -> (-245.175, 74.7758) centre (-244.4679, 75.4829) ccw
  line L19 (-242, 106.095) -> (-242, 95.905)
  line L20 (-245.175, 87.2242) -> (-245.175, 94.7758)
  line L21 (-242, 86.095) -> (-243.5613, 86.095)
  line L22 (-243.5613, 95.905) -> (-242, 95.905)
  arc A9 (-245.175, 87.2242) -> (-243.5613, 86.095) centre (-244.4679, 86.5171) ccw
  arc A10 (-243.5613, 95.905) -> (-245.175, 94.7758) centre (-244.4679, 95.4829) ccw
  line L23 (-245.175, 0) -> (-246.905, 0)
  line L24 (-302, 182) -> (-242, 182) construction
  line L25 (-242, 182) -> (-242, 0) construction
  line L26 (-242, 0) -> (-302, 0) construction
  line L27 (-302, 0) -> (-302, 182) construction
  line L28 (-272, 182) -> (-272, 10.7369) construction
  arc A11 (-298.825, 14.7758) -> (-300.4387, 15.905) centre (-299.5321, 15.4829) ccw
  arc A12 (-300.4387, 26.095) -> (-298.825, 27.2242) centre (-299.5321, 26.5171) ccw
  line L29 (-302, 46.095) -> (-302, 35.905)
  line L30 (-300.4387, 35.905) -> (-302, 35.905)
  arc A13 (-298.825, 34.7758) -> (-300.4387, 35.905) centre (-299.5321, 35.4829) ccw
  line L31 (-298.825, 27.2242) -> (-298.825, 34.7758)
  line L32 (-298.825, 0) -> (-298.825, 14.7758)
  line L33 (-302, 26.095) -> (-302, 15.905)
  line L34 (-300.4387, 15.905) -> (-302, 15.905)
  line L35 (-302, 26.095) -> (-300.4387, 26.095)
  line L36 (-302, 66.095) -> (-302, 55.905)
  line L37 (-300.4387, 55.905) -> (-302, 55.905)
  line L38 (-298.825, 47.2242) -> (-298.825, 54.7758)
  line L39 (-302, 46.095) -> (-300.4387, 46.095)
  arc A14 (-300.4387, 46.095) -> (-298.825, 47.2242) centre (-299.5321, 46.5171) ccw
  arc A15 (-298.825, 54.7758) -> (-300.4387, 55.905) centre (-299.5321, 55.4829) ccw
  line L40 (-302, 86.095) -> (-302, 75.905)
  line L41 (-300.4387, 75.905) -> (-302, 75.905)
  line L42 (-298.825, 67.2242) -> (-298.825, 74.7758)
  line L43 (-302, 66.095) -> (-300.4387, 66.095)
  arc A16 (-300.4387, 66.095) -> (-298.825, 67.2242) centre (-299.5321, 66.5171) ccw
  arc A17 (-298.825, 74.7758) -> (-300.4387, 75.905) centre (-299.5321, 75.4829) ccw
  line L44 (-302, 106.095) -> (-302, 95.905)
  line L45 (-300.4387, 95.905) -> (-302, 95.905)
  line L46 (-298.825, 87.2242) -> (-298.825, 94.7758)
  line L47 (-302, 86.095) -> (-300.4387, 86.095)
  arc A18 (-300.4387, 86.095) -> (-298.825, 87.2242) centre (-299.5321, 86.5171) ccw
  arc A19 (-298.825, 94.7758) -> (-300.4387, 95.905) centre (-299.5321, 95.4829) ccw
  line L48 (-298.825, 0) -> (-286.905, 0)
  line L49 (-302, 91) -> (-242, 91) construction
  arc A20 (-300.4387, 166.095) -> (-298.825, 167.2242) centre (-299.5321, 166.5171) ccw
  line L50 (-300.4387, 166.095) -> (-302, 166.095)
  line L51 (-298.825, 182) -> (-298.825, 167.2242)
  line L52 (-243.5613, 166.095) -> (-242, 166.095)
  line L53 (-245.175, 182) -> (-245.175, 167.2242)
  arc A21 (-245.175, 167.2242) -> (-243.5613, 166.095) centre (-244.4679, 166.5171) ccw
  line L54 (-245.175, 182) -> (-246.905, 182)
  line L55 (-285.7758, 178.825) -> (-278.2242, 178.825)
  line L56 (-277.095, 180.4387) -> (-277.095, 182)
  arc A22 (-278.2242, 178.825) -> (-277.095, 180.4387) centre (-277.5171, 179.5321) ccw
  line L57 (-286.905, 182) -> (-286.905, 180.4387)
  line L58 (-298.825, 182) -> (-286.905, 182)
  arc A23 (-286.905, 180.4387) -> (-285.7758, 178.825) centre (-286.4829, 179.5321) ccw
  line L59 (-266.905, 182) -> (-277.095, 182)
  line L60 (-242, 126.095) -> (-242, 115.905)
  line L61 (-245.175, 107.2242) -> (-245.175, 114.7758)
  line L62 (-242, 106.095) -> (-243.5613, 106.095)
  line L63 (-243.5613, 115.905) -> (-242, 115.905)
  arc A24 (-245.175, 107.2242) -> (-243.5613, 106.095) centre (-244.4679, 106.5171) ccw
  arc A25 (-243.5613, 115.905) -> (-245.175, 114.7758) centre (-244.4679, 115.4829) ccw
  line L64 (-242, 146.095) -> (-242, 135.905)
  line L65 (-245.175, 127.2242) -> (-245.175, 134.7758)
  line L66 (-242, 126.095) -> (-243.5613, 126.095)
  line L67 (-243.5613, 135.905) -> (-242, 135.905)
  arc A26 (-245.175, 127.2242) -> (-243.5613, 126.095) centre (-244.4679, 126.5171) ccw
  arc A27 (-243.5613, 135.905) -> (-245.175, 134.7758) centre (-244.4679, 135.4829) ccw
  line L68 (-242, 166.095) -> (-242, 155.905)
  line L69 (-245.175, 147.2242) -> (-245.175, 154.7758)
  line L70 (-242, 146.095) -> (-243.5613, 146.095)
  line L71 (-243.5613, 155.905) -> (-242, 155.905)
  arc A28 (-245.175, 147.2242) -> (-243.5613, 146.095) centre (-244.4679, 146.5171) ccw
  arc A29 (-243.5613, 155.905) -> (-245.175, 154.7758) centre (-244.4679, 155.4829) ccw
  arc A30 (-265.7758, 3.175) -> (-266.905, 1.5613) centre (-266.4829, 2.4679) ccw
  line L72 (-265.7758, 3.175) -> (-258.2242, 3.175)
  line L73 (-246.905, 0) -> (-257.095, 0)
  line L74 (-266.905, 0) -> (-266.905, 1.5613)
  line L75 (-257.095, 1.5613) -> (-257.095, 0)
  arc A31 (-257.095, 1.5613) -> (-258.2242, 3.175) centre (-257.5171, 2.4679) ccw
  line L76 (-302, 126.095) -> (-302, 115.905)
  line L77 (-300.4387, 115.905) -> (-302, 115.905)
  line L78 (-298.825, 107.2242) -> (-298.825, 114.7758)
  line L79 (-302, 106.095) -> (-300.4387, 106.095)
  arc A32 (-300.4387, 106.095) -> (-298.825, 107.2242) centre (-299.5321, 106.5171) ccw
  arc A33 (-298.825, 114.7758) -> (-300.4387, 115.905) centre (-299.5321, 115.4829) ccw
  line L80 (-302, 146.095) -> (-302, 135.905)
  line L81 (-300.4387, 135.905) -> (-302, 135.905)
  line L82 (-298.825, 127.2242) -> (-298.825, 134.7758)
  line L83 (-302, 126.095) -> (-300.4387, 126.095)
  arc A34 (-300.4387, 126.095) -> (-298.825, 127.2242) centre (-299.5321, 126.5171) ccw
  arc A35 (-298.825, 134.7758) -> (-300.4387, 135.905) centre (-299.5321, 135.4829) ccw
  line L84 (-302, 166.095) -> (-302, 155.905)
  line L85 (-300.4387, 155.905) -> (-302, 155.905)
  line L86 (-298.825, 147.2242) -> (-298.825, 154.7758)
  line L87 (-302, 146.095) -> (-300.4387, 146.095)
  arc A36 (-300.4387, 146.095) -> (-298.825, 147.2242) centre (-299.5321, 146.5171) ccw
  arc A37 (-298.825, 154.7758) -> (-300.4387, 155.905) centre (-299.5321, 155.4829) ccw
  arc A38 (-266.905, 180.4387) -> (-265.7758, 178.825) centre (-266.4829, 179.5321) ccw
  line L88 (-257.095, 180.4387) -> (-257.095, 182)
  line L89 (-246.905, 182) -> (-257.095, 182)
  line L90 (-265.7758, 178.825) -> (-258.2242, 178.825)
  line L91 (-266.905, 182) -> (-266.905, 180.4387)
  arc A39 (-258.2242, 178.825) -> (-257.095, 180.4387) centre (-257.5171, 179.5321) ccw
  point P0 (-302, 0)
  point P1 (-266.095, 0)
  point P2 (-302, 182)
  point P3 (-266.095, 182)
  point P4 (-302, 182)
  point P5 (-242, 182)
  point P6 (-277.905, 182)
  point P7 (-285.905, 180.4387)
  point P8 (-284.7758, 178.825)
  point P9 (-285.4829, 179.5321)
  point P10 (-285.905, 182)
  point P11 (-302, 182)
  point P12 (-302, 182)
  point P13 (-266.095, 182)
  point P14 (-265.905, 180.4387)
  point P15 (-252, 182)
  point P16 (-264.7758, 178.825)
  point P17 (-265.905, 182)
  point P18 (-265.4829, 179.5321)
  dimension "d1887" = 2
  dimension "d1888" = 0.4221
  dimension "d1889" = 0.7071
  dimension "d1890" = 0.4221
  dimension "d1896" = 2
  dimension "d1899" = 2
  dimension "d1926" = 3.175
  dimension "d1948" = 0.7071
  dimension "d1949" = 0.4221
  dimension "d1951" = 0.4221
  dimension "d1953" = 9.81
  dimension "d1956" = 10.19
  dimension "d1958" = 0.4221
  dimension "d1959" = 0.7071
  dimension "d1960" = 0.7071
  dimension "d1961" = 9.81
  dimension "d1962" = 10.19
  dimension "d1963" = 242
  dimension "d1965" = 3.175
  dimension "d1975" = 15.905
  dimension "d1976" = 10.19
  dimension "d1992" = 20
  dimension "d1993" = 20
  dimension "d2004" = 20
  dimension "d2005" = 0
  dimension "d2012" = 1.73
  dimension "d2140" = 60
  dimension "d2141" = 182
  dimension "d2142" = 242
  dimension "d2145" = 15.095
  dimension "d2148" = 0
  dimension "d2149" = 20
  dimension "d2152" = 20
  dimension "d2153" = 0
  constraint horizontal L9
  constraint perpendicular L0 L3
  constraint perpendicular L3 L4
  constraint equal A3 A4
  constraint horizontal A4.centre A3.centre
  constraint perpendicular L1 L9
  constraint equal A1 A2
  constraint coincident L0.start L9
  constraint perpendicular L6 L7
  constraint perpendicular L5 L10
  constraint vertical L8
  constraint collinear L1 L8
  constraint collinear L6 L10
  constraint coincident L1 L23.start
  constraint perpendicular L1 L23
  constraint coincident L1.start L23.start
  constraint horizontal L24
  constraint vertical L25
  constraint horizontal L26
  constraint vertical L27
  constraint midpoint L24 L28.start
  constraint perpendicular L26 L28
  constraint coincident origin L26
  constraint symmetric L5.end L28 L33.end
  constraint symmetric L2.end L28 L29.end
  constraint symmetric L6.start L28 L33.start
  constraint symmetric L1.start L28 L32.start
  constraint symmetric L1.end L28 A11.start
  constraint symmetric L5.start L28 A11.end
  constraint symmetric A0 L28 A11
  constraint symmetric A1.end L28 A12.start
  constraint symmetric A1.start L28 A12.end
  constraint symmetric A1 L28 A12
  constraint symmetric L8.end L28 A13.start
  constraint symmetric L2.start L28 L30.start
  constraint symmetric A2 L28 A13
  constraint symmetric L10.start L28 L29.start
  constraint symmetric L25.end L28 P0
  constraint perpendicular L0 L48
  constraint midpoint L27 L49.start
  constraint midpoint L25 L49.end
  constraint coincident L48 origin
  constraint symmetric P0 L49 P12
  constraint symmetric L33.end L49 L50.end
  constraint symmetric P1 L49 P13
  constraint symmetric A11.start L49 A20.end
  constraint symmetric A11.end L49 A20.start
  constraint symmetric L32.start L49 L51.start
  constraint symmetric A11 L49 A20
  constraint symmetric L5.end L49 L52.end
  constraint symmetric L1.start L49 L53.start
  constraint symmetric L1.end L49 L53.end
  constraint symmetric L5.start L49 L52.start
  constraint symmetric A0 L49 A21
  constraint symmetric L23.end L49 L54.end
  constraint symmetric L25.end L49 P5
  constraint symmetric L0.start L49 L57.start
  constraint symmetric L4.end L49 L56.end
  constraint symmetric L0.end L49 L57.end
  constraint symmetric L3.start L49 L55.start
  constraint symmetric A3 L49 A23
  constraint symmetric L3.end L49 L55.end
  constraint symmetric L4.start L49 L56.start
  constraint symmetric A4 L49 A22
  constraint symmetric L9.start L49 L59.start
  measures "d1887" diameter of A3
  measures "d1888" distance of A3.centre L0
  measures "d1889" distance of A3.centre L3
  measures "d1890" horizontal distance of A4.centre L4.end
  measures "d1896" diameter of A1
  measures "d1899" diameter of A0
  measures "d1926" distance of L3 L9
  measures "d1948" distance of A0.centre L1
  measures "d1949" distance of A0.centre L5
  measures "d1951" distance of A1.centre L7
  measures "d1953" distance of L2 L7
  measures "d1956" distance of L5 A1.end
  measures "d1958" distance of A2.centre L2
  measures "d1959" distance of A1.centre L8
  measures "d1960" distance of A2.centre L8
  measures "d1961" distance of L0 L4
  measures "d1962" distance of L2 L10.start
  measures "d1963" distance of origin L6
  measures "d1965" distance of L6 L8
  measures "d1975" distance of L1.start L5
  measures "d1976" distance of L4.end L9.start
  measures "d2012" distance of L1.start L23.end
  measures "d2140" distance of P12 P5
  measures "d2141" distance of P12 P0
  measures "d2142" horizontal distance of origin L25.end
  measures "d2145" distance of L0 P0
extrude "Extrude22" add sketch "MyStock" along normal blind 3.175 separate body makes body 2
equation "fingerWidth = 10 mm"
equation "length = 240 mm"
equation "thickness = 3.175 mm"
equation "height = 60 mm"
equation "toolDiameter = 2 mm"
equation "d34 = toolDiameter"
equation "d36 = boneCenterToHoleSide"
equation "d37 = boneCenterToHoleBottom"
equation "d38 = boneCenterToHoleSide"
equation "boneCenterToHoleBottom = toolDiameter / 2 / sqrt(2) - 0 * kerf" comment "Best: 2.001 -2*kerf, 0.1;;;Best: 2.001 no kerf and 0.1   OLD+6 kerf at 2.001 Diam and .1 mm"
equation "tempLengthPieces = ceil(( ( floor(( length - 2 * thickness ) / fingerWidth) - 2 ) - ( ( floor(( length - 2 * thickness ) / fingerWidth) - 2 ) % 2 - 1 ) ))"
equation "lengthCuts = ceil(tempLengthPieces / 2)"
equation "shoulderToothLength = ( length - fingerWidth * tempLengthPieces ) / 2 - kerf"
equation "depth = 182 mm"
equation "tempDepthPieces = ceil(( ( floor(( depth - 2 * thickness ) / fingerWidth) - 2 ) - ( ( floor(( depth - 2 * thickness ) / fingerWidth) - 2 ) % 2 - 1 ) ))"
equation "depthCuts = ceil(tempDepthPieces / 2)"
equation "shoulderToothDepth = ( depth - fingerWidth * tempDepthPieces ) / 2 - kerf"
equation "d48 = toolDiameter"
equation "d49 = boneCenterToHoleSide"
equation "d50 = shoulderToothDepth"
equation "d52 = boneCenterToHoleSide"
equation "d54 = boneCenterToHoleBottom"
equation "d55 = holeWidth"
equation "tempHeightPieces = ceil(( ( floor(( height - 2 * thickness ) / fingerWidth) - 2 ) - ( ( floor(( height - 2 * thickness ) / fingerWidth) - 2 ) % 2 - 1 ) ))"
equation "heightCuts = ceil(tempHeightPieces / 2)"
equation "sholderToothHeight = ( height - fingerWidth * tempHeightPieces ) / 2 - kerf"
equation "d189 = shoulderToothLength"
equation "kerf = -0.095 mm"
equation "holeWidth = fingerWidth + 2 * kerf"
equation "shoulderHoleLength = shoulderToothLength + 2 * kerf"
equation "shouderHoleDepth = shoulderToothDepth + 2 * kerf"
equation "shoulderHoleHeight = sholderToothHeight + 2 * kerf"
equation "assembleScrewDiam = 2.1 mm"
equation "assembleScrewDistance = 6 mm"
equation "assembleAvoidCollisionDistance = 1 mm"
equation "coolingHoleDistance = 8 mm"
equation "boneCornerToCenterPack = -3 * kerf"
equation "boneCenterToHoleSide = boneCenterToHoleBottom - boneCornerToCenterPack"
equation "d473 = length"
equation "d479 = -toolDiameter / 2"
equation "pumpLength = 52 mm"
equation "pumpCircleDiam = 30 mm"
equation "pumpHeight = 34 mm"
equation "sensorWireDistance = 10 mm"
equation "sensorWireDiam = 3.5 mm"
equation "pumpScrewDiam = 3 mm"